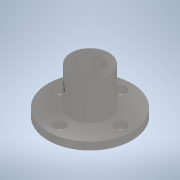
# Autodesk Inventor part: 9_Flangia
Saved by Autodesk Inventor 2020.2 (Build 242310000, 310)
## iProperties
Created: 2019-10-15
Part Number: 9_Flangia
Material: Acciaio, Dolce
Document SubType Name: Modeling
Designer: socci
Density: 7.85 g/cm^3
Appearance: Semilucidato
Mass: 10.2775 g
Surface Area: 13.859 cm^2
Volume: 1.30924 cm^3
Author: socci
Autodesk Inventor part; units mm, degrees
ref_plane "YZ Plane" through (0, 0, 0) normal (1, 0, 0) x (0, 1, 0)
ref_plane "XZ Plane" through (0, 0, 0) normal (0, 1, 0) x (-1, 0, 0)
ref_plane "XY Plane" through (0, 0, 0) normal (0, 0, 1) x (1, 0, 0)
sketch "Schizzo1" plane through (0, 0, 0) normal (0, 1, 0) x (-1, 0, 0)
  circle A0 centre (0, 0) radius 11
  dimension "d0" = 22
  constraints: 1 centre point, 1 coincident
  measures "d0" diameter of A0
extrude "Estrusione1" add sketch "Schizzo1" along normal blind 2
sketch "Schizzo2" plane through (0, 2, 0) normal (0, 1, 0) x (1, 0, 0)
  circle A0 centre (0, 0) radius 5
  line L0 (-7, -1) -> (-1, 7)
  line L1 (-1, 7) -> (7, 1)
  line L2 (7, 1) -> (1, -7)
  line L3 (1, -7) -> (-7, -1)
  point P0 (-3, -4)
  point P1 (4, -3)
  point P2 (-4, 3)
  point P3 (3, 4)
  dimension "d3" = 10
  constraints: 8 end point, 2 coincident, 1 midpoint, 12 other
extrude "Estrusione2" add sketch "Schizzo2" along normal blind 10
sketch "Schizzo3" plane through (0, 0, 0) normal (0, -1, 0) x (1, 0, 0)
  circle A0 centre (0, 0) radius 2
  circle A1 centre (-8, 0) radius 1.5
  line L0 (0, -8) -> (0, 8)
  line L1 (-8, 0) -> (8, 0)
  circle A2 centre (0, -8) radius 1.5
  circle A3 centre (8, 0) radius 1.5
  circle A4 centre (0, 8) radius 1.5
  dimension "d6" = 4
  dimension "d7" = 3
  dimension "d8" = 16
  dimension "d9" = 16
  dimension "d10" = 3
  dimension "d11" = 3
  dimension "d12" = 3
  constraints: 6 coincident, 5 centre point, 4 end point, 2 midpoint, 1 perpendicular, 1 vertical
  measures "d6" diameter of A0
  measures "d7" diameter of A1
  measures "d8" distance of L0.start L0.end
  measures "d9" distance of L1.start L1.end
  measures "d10" diameter of A2
  measures "d11" diameter of A3
  measures "d12" diameter of A4
extrude "Estrusione3" cut sketch "Schizzo3" against normal blind 2 contours A2 | A1 | A4 | A3
sketch "Schizzo4" plane through (0, 0, 0) normal (0, -1, 0) x (1, 0, 0)
  circle A0 centre (0, 0) radius 3
  dimension "d15" = 6
  constraints: 1 centre point, 1 coincident
  measures "d15" diameter of A0
extrude "Estrusione4" cut sketch "Schizzo4" against normal blind 12
sketch "Schizzo5" plane through (1, 2, 7) normal (-0.6, 0, 0.8) x (0.8, 0, 0.6)
  line L0 (-0.7385, 0) -> (-9.9134, 0) projected
  line L1 (-5, 0) -> (-5, 4)
  line L2 (-5, 0) -> (-1, 0) construction
  line L3 (-5, 4) -> (-5, 5.5)
  point P0 (-5, -2)
  dimension "d19" = 4
  dimension "d20" = 90
  dimension "d21" = 1.5
  dimension "d22" = 180
  constraints: 6 end point, 2 perpendicular, 1 collinear, 1 horizontal, 1 point on line
  measures "d19" distance of L1.start L1.end
  measures "d20" angle of L2 L1
  measures "d21" distance of L1.end L3.end
  measures "d22" angle of L3 L1
hole "Foro1" at (-3, 7.5, 4) direction (0.6, 0, -0.8) diameter 2.459 depth 6 tip angle 118 thread size "M3x0.5" class "6H" standard "ISO Metric profile"
sketch "Schizzo7" plane through (-1, 2, -7) normal (0.6, 0, -0.8) x (-0.8, 0, -0.6)
  circle A0 centre (-5, 5.5) radius 1.2295 projected
  circle A1 centre (-5, 5.5) radius 1.2295
  point P0 (-5, -2)
  point P1 (-6.2295, 5.5)
  constraints: 1 centre point, 1 coincident, 1 horizontal alignment, 1 other
hole "Foro2" at (3, 7.5, -4) direction (-0.6, 0, 0.8) diameter 2.459 depth 6 tip angle 118 thread size "M3x0.5" class "6H" standard "ISO Metric profile"
sketch "Schizzo6" plane through (0, 12, 0) normal (0, 1, 0) x (1, 0, 0)
  circle A0 centre (0, 0) radius 5
  circle A1 centre (0, 0) radius 3 projected
  line L0 (-1, 7) -> (-7, -1) projected
  line L1 (-1, 7) -> (7, 1)
  line L2 (7, 1) -> (1, -7)
  line L3 (1, -7) -> (-7, -1)
  line L4 (-7, -1) -> (-1, 7)
  point P0 (-4, 3)
  point P1 (-3, -4)
  point P2 (4, -3)
  point P3 (-4, 3)
  point P4 (3, 4)
  constraints: 8 end point, 2 coincident, 2 midpoint, 1 centre point, 9 other
extrude "Estrusione5" cut sketch "Schizzo6" against normal blind 10 contours A0 L1 L2 | A0 L0 L1 | L2 L3 A0 | A0 L3 L0
